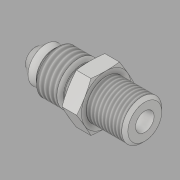
# Autodesk Inventor part: AN816-4D
Saved by Autodesk Inventor 2019 (Build 230136000, 136)
## iProperties
Created: 2018-11-23
Part Number: AN816-4D
Material: Aluminum 2014-T6
Document SubType Name: Modeling
Designer: erics
Density: 2.78927 g/cm^3
Appearance: Satin
Mass: 5.55221 g
Surface Area: 15.5407 cm^2
Volume: 1.99056 cm^3
Author: erics
Autodesk Inventor part; units mm, degrees
ref_plane "YZ Plane" through (0, 0, 0) normal (1, 0, 0) x (0, 1, 0)
ref_plane "XZ Plane" through (0, 0, 0) normal (0, 1, 0) x (-1, 0, 0)
ref_plane "XY Plane" through (0, 0, 0) normal (0, 0, 1) x (1, 0, 0)
sketch "Sketch4" plane through (0, 0, 0) normal (0, 0, 1) x (1, 0, 0)
  line L0 (0, 0) -> (0, 2.4511)
  line L1 (0.0506, 2.5525) -> (2.7136, 4.5593)
  line L2 (2.7136, 4.5593) -> (4.797, 4.5593)
  line L3 (4.9766, 4.6337) -> (5.8991, 5.5563)
  line L4 (5.8991, 5.5563) -> (11.1316, 5.5563)
  line L5 (11.1316, 5.5563) -> (11.9906, 4.6972)
  line L6 (12.1702, 4.6228) -> (13.97, 4.6228)
  line L7 (13.97, 4.6228) -> (13.97, 0)
  line L8 (13.97, 0) -> (0, 0)
  arc A0 (0.0506, 2.5525) -> (0, 2.4511) centre (0.127, 2.4511) ccw
  arc A1 (4.797, 4.5593) -> (4.9766, 4.6337) centre (4.797, 4.8133) ccw
  arc A2 (11.9906, 4.6972) -> (12.1702, 4.6228) centre (12.1702, 4.8768) ccw
  point P0 (4.9022, 4.5593)
  point P1 (12.065, 4.6228)
  dimension "d26" = 45
  dimension "d28" = 13.97
  dimension "d29" = 0.127
  dimension "d30" = 2.4511
  dimension "d31" = 37
  dimension "d32" = 4.9022
  dimension "d33" = 4.5593
  dimension "d34" = 0.254
  dimension "d35" = 4.6228
  dimension "d36" = 5.5563
  dimension "d37" = 45
  dimension "d39" = 1.905
  constraints: 18 end point, 6 point on circle, 6 tangent, 4 point on line, 3 centre point, 3 perpendicular, 1 equal radius, 1 parallel, 1 vertical
  measures "d26" angle of L4 L3
  measures "d28" distance between parallel lines of L7 L0
  measures "d29" radius of A0
  measures "d30" distance of L0.start L0.end
  measures "d31" angle of L2 L1
  measures "d32" distance from line of L0 point (4.902, 4.559)
  measures "d33" distance between parallel lines of L8 L2
  measures "d34" radius of A1
  measures "d35" distance of L6.end L7.end
  measures "d36" distance between parallel lines of L8 L4
  measures "d37" angle of L4 L5
  measures "d39" distance from line of L7 point (12.065, 4.623)
revolve "Revolution3" add sketch "Sketch4" angle 360 about axis through (13.97, 0, 0) along (-1, 0, 0)
sketch "Sketch5" plane through (13.97, 8.382, 0) normal (-1, 0, 0) x (0, -1, 0)
  line L0 (2.032, 3.6662) -> (8.382, 7.3323)
  line L1 (8.382, 7.3323) -> (14.732, 3.6662)
  line L2 (14.732, 3.6662) -> (14.732, -3.6662)
  line L3 (14.732, -3.6662) -> (8.382, -7.3323)
  line L4 (8.382, -7.3323) -> (2.032, -3.6662)
  line L5 (2.032, -3.6662) -> (2.032, 3.6662)
  circle A0 centre (8.382, 0) radius 7.3323 construction
  point P0 (8.382, 0)
  dimension "d42" = 14.6647
  dimension "d41" = 12.7
  constraints: 12 end point, 2 coincident, 1 vertical, 16 other
  measures "d41" distance between parallel lines of L2 L5
extrude "Extrusion2" add sketch "Sketch5" against normal blind 4.2672
sketch "Sketch9" plane through (18.2372, 8.382, 0) normal (1, 0, 0) x (0, 0, -1)
  circle A0 centre (0, -8.382) radius 5.1435
  dimension "d66" = 10.287
  constraints: 1 centre point, 1 coincident
  measures "d66" diameter of A0
extrude "Extrusion3" add sketch "Sketch9" along normal blind 9.9314
chamfer "Chamfer1" distance 0.7874 angle 45 1 edges at (28.1686, 0, 5.1435)
thread "Thread2" size "1/8" designation "1/8 - 27 NPT" standard "NPT" full length
sketch "Sketch7" plane through (0, 0, 0) normal (-1, 0, 0) x (0, 0, 1)
  circle A0 centre (0, 0) radius 2.4511 projected
  point P0 (0, 0)
  constraints: 1 coincident
hole "Hole1" at (0, 0, 0) direction (1, 0, 0) diameter 4.3688 depth 13.97 tip angle 118 start extended yes
thread "Thread3" size "7/16-20 UNF" class "3A" standard "ANSI Unified Screw Threads" full length
sketch "Sketch8" plane through (0, 0, 0) normal (0, 1, 0) x (-1, 0, 0)
  line L0 (-12.1702, 4.6228) -> (-13.97, 4.6228) construction
  line L1 (-13.97, 3.6662) -> (-13.97, 7.3323) construction
  line L2 (-13.97, 3.6662) -> (-13.97, 7.3323) construction
  line L3 (-13.97, 7.3323) -> (-18.2372, 7.3323) construction
  line L4 (-18.2372, 3.6662) -> (-18.2372, 7.3323) construction
  line L5 (-13.97, 3.6662) -> (-18.2372, 3.6662) construction
  line L6 (-14.2332, 7.3323) -> (-13.97, 6.35)
  line L7 (-14.2332, 7.3323) -> (-13.97, 7.3323)
  line L8 (-13.97, 6.35) -> (-13.97, 7.3323)
  line L9 (-16.1036, 7.3323) -> (-16.1036, 3.6662)
  line L10 (-13.97, 3.6662) -> (-18.2372, 3.6662) projected
  line L11 (-17.974, 7.3323) -> (-18.2372, 6.35)
  line L12 (-17.974, 7.3323) -> (-18.2372, 7.3323)
  line L13 (-18.2372, 6.35) -> (-18.2372, 7.3323)
  line L14 (5.9538, 0) -> (-35.7226, 0) projected
  point P0 (0, 0)
  point P1 (-18.2372, 7.3323)
  dimension "d62" = 6.35
  dimension "d64" = 15
  constraints: 14 end point, 4 symmetric about line, 2 midpoint, 2 point on line, 1 collinear, 1 perpendicular
  measures "d62" vertical distance of L6.end point (0, 0)
  measures "d64" angle of L1 L6
revolve "Revolution5" cut sketch "Sketch8" angle 360 about axis through (-10, 0, 0) along (1, 0, 0)
sketch "Sketch10" plane through (28.1686, 0, 0) normal (1, 0, 0) x (0, 0, -1)
  circle A0 centre (0, 0) radius 4.3561 projected
  constraints: 1 coincident
hole "Hole2" at (28.1686, 0, 0) direction (-1, 0, 0) diameter 4.7752 depth 14.1986 tip angle 118 start extended yes
equation "\"d28\" = MS33656_J"
equation "\"d30\" = 0.5 * MS33656_D"
equation "\"d32\" = MS33656_B"
equation "\"d33\" = 0.5 * MS33656_C"
equation "\"d35\" = 0.5 * MS33656_F"
equation "\"d36\" = 0.5 * AN816_T"
equation "\"d39\" = MS33656_Q"
equation "\"d41\" = AN816_G"
equation "\"d44\" = -MS33656_J + AN816_M - MS33677_F"
equation "\"d66\" = MS33677_D"
equation "\"d67\" = MS33677_F"
equation "\"d69\" = MS33677_J"
equation "\"d53\" = MS33656_A"
equation "\"d62\" = 0.5 * AN816_G"
equation "\"d72\" = MS33677_G"
equation "\"AN816_T\" = 11.1125"
equation "\"AN816_G\" = 12.7"
equation "\"AN816_M\" = 28.1686"
equation "\"MS33656_A\" = 4.3688"
equation "\"MS33656_D\" = 4.9022"
equation "\"MS33656_B\" = 4.9022"
equation "\"MS33656_C\" = 9.1186"
equation "\"MS33656_F\" = 9.2456"
equation "\"MS33656_J\" = 13.97"
equation "\"MS33656_Q\" = 1.905"
equation "\"MS33677_F\" = 9.9314"
equation "\"MS33677_D\" = 10.287"
equation "\"MS33677_J\" = 0.7874"
equation "\"MS33677_C\" = 11.9126"
equation "\"MS33677_G\" = 4.7752"
body "Solid2"
